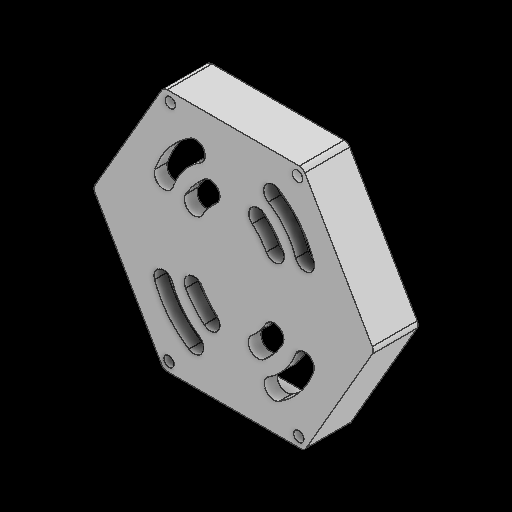
# Autodesk Inventor part: ArmPowerBoardBack
Saved by Autodesk Inventor 2025.2 (Build 292293000, 293)
## iProperties
Created: 2026-06-24
Part Number: ArmPowerBoardBack
Material: Generic
Document SubType Name: Modeling
Designer: valer
Density: 1 g/cm^3
Appearance: Default
Author: valer
Autodesk Inventor part; units mm, degrees
ref_plane "YZ Plane" through (0, 0, 0) normal (1, 0, 0) x (0, 1, 0)
ref_plane "XZ Plane" through (0, 0, 0) normal (0, 1, 0) x (-1, 0, 0)
ref_plane "XY Plane" through (0, 0, 0) normal (0, 0, 1) x (1, 0, 0)
sketch "Sketch1" plane through (0, 0, 0) normal (0, 0, 1) x (1, 0, 0)
  circle A0 centre (-20.1638, -35.1051) radius 1.25 projected
  circle A1 centre (19.9556, 35.1051) radius 1.25 projected
  circle A2 centre (20.3721, -35.1051) radius 1.25 projected
  circle A3 centre (-19.7473, 35.1051) radius 1.25 projected
  arc A4 (-17.1638, -35.1051) -> (-21.6638, -32.507) centre (-20.1638, -35.1051) ccw projected
  arc A5 (-23.0299, -32.141) -> (-21.6638, -32.507) centre (-22.1638, -31.641) ccw projected
  line L0 (-23.0299, -32.141) -> (-41.5865, 0) projected
  line L1 (-41.5865, 0) -> (-22.9176, 32.3355) projected
  arc A6 (-21.4755, 32.6529) -> (-22.9176, 32.3355) centre (-22.0516, 31.8355) ccw projected
  arc A7 (-21.4755, 32.6529) -> (-16.7473, 35.1051) centre (-19.7473, 35.1051) ccw projected
  arc A8 (-15.7473, 36.1051) -> (-16.7473, 35.1051) centre (-15.7473, 35.1051) ccw projected
  line L2 (-15.7473, 36.1051) -> (15.9556, 36.1051) projected
  arc A9 (16.9556, 35.1051) -> (15.9556, 36.1051) centre (15.9556, 35.1051) ccw projected
  arc A10 (16.9556, 35.1051) -> (21.4556, 32.507) centre (19.9556, 35.1051) ccw projected
  arc A11 (22.8216, 32.141) -> (21.4556, 32.507) centre (21.9556, 31.641) ccw projected
  line L3 (22.8216, 32.141) -> (41.5865, -0.3607) projected
  line L4 (41.5865, -0.3607) -> (23.2381, -32.141) projected
  arc A12 (21.8721, -32.507) -> (23.2381, -32.141) centre (22.3721, -31.641) ccw projected
  arc A13 (21.8721, -32.507) -> (17.3721, -35.1051) centre (20.3721, -35.1051) ccw projected
  arc A14 (16.3721, -36.1051) -> (17.3721, -35.1051) centre (16.3721, -35.1051) ccw projected
  line L5 (16.3721, -36.1051) -> (-16.1638, -36.1051) projected
  arc A15 (-17.1638, -35.1051) -> (-16.1638, -36.1051) centre (-16.1638, -35.1051) ccw projected
  line L6 (-43.3185, -1) -> (-22.4732, -37.1051) projected
  arc A16 (-22.4732, -37.1051) -> (-20.7412, -38.1051) centre (-20.7412, -36.1051) ccw projected
  line L7 (-20.7412, -38.1051) -> (20.9494, -38.1051) projected
  arc A17 (20.9494, -38.1051) -> (22.6815, -37.1051) centre (20.9494, -36.1051) ccw projected
  line L8 (22.6815, -37.1051) -> (43.3185, -1.3607) projected
  arc A18 (43.3185, -1.3607) -> (43.3185, 0.6393) centre (41.5865, -0.3607) ccw projected
  line L9 (43.3185, 0.6393) -> (22.265, 37.1051) projected
  arc A19 (22.265, 37.1051) -> (20.5329, 38.1051) centre (20.5329, 36.1051) ccw projected
  line L10 (20.5329, 38.1051) -> (-20.7412, 38.1051) projected
  arc A20 (-20.7412, 38.1051) -> (-22.4732, 37.1051) centre (-20.7412, 36.1051) ccw projected
  line L11 (-22.4732, 37.1051) -> (-43.3185, 1) projected
  arc A21 (-43.3185, 1) -> (-43.3185, -1) centre (-41.5865, 0) ccw projected
  point P0 (0, 0)
extrude "Extrusion1" add sketch "Sketch1" along normal blind 10
sketch "Sketch2" plane through (0, 0, 10) normal (0, 0, 1) x (1, 0, 0)
  arc A0 (19.392, 12.5813) -> (25.0985, 14.4351) centre (22.2452, 13.5082) ccw projected
  arc A1 (19.392, 12.5813) -> (10.8356, 23.4883) centre (0.2256, 6.3551) ccw projected
  arc A2 (13.9946, 28.5893) -> (10.8356, 23.4883) centre (12.4151, 26.0388) ccw projected
  arc A3 (25.0985, 14.4351) -> (13.9946, 28.5893) centre (0.2256, 6.3551) ccw projected
  arc A4 (-19.0054, -13.2092) -> (-24.656, -15.2268) centre (-21.8307, -14.218) ccw projected
  arc A5 (-19.0054, -13.2092) -> (-10.7215, -23.5712) centre (0.1909, -6.3551) ccw projected
  arc A6 (-13.9337, -28.639) -> (-10.7215, -23.5712) centre (-12.3276, -26.1051) ccw projected
  arc A7 (-24.656, -15.2268) -> (-13.9337, -28.639) centre (0.1909, -6.3551) ccw projected
  arc A8 (10.216, 9.6769) -> (15.4555, 12.6005) centre (12.8358, 11.1387) ccw projected
  arc A9 (10.216, 9.6769) -> (5.8047, 15.0962) centre (-7.382, -0.1428) ccw projected
  arc A10 (9.7308, 19.6334) -> (5.8047, 15.0962) centre (7.7677, 17.3648) ccw projected
  arc A11 (15.4555, 12.6005) -> (9.7308, 19.6334) centre (-7.382, -0.1428) ccw projected
  arc A12 (-5.3056, 15.1266) -> (-9.2069, 19.6851) centre (-7.2562, 17.4058) ccw projected
  arc A13 (-5.3056, 15.1266) -> (-9.7465, 9.7314) centre (7.7976, -0.1843) ccw projected
  arc A14 (-14.9699, 12.6837) -> (-9.7465, 9.7314) centre (-12.3582, 11.2076) ccw projected
  arc A15 (-9.2069, 19.6851) -> (-14.9699, 12.6837) centre (7.7976, -0.1843) ccw projected
  arc A16 (-9.7465, -9.7314) -> (-14.9699, -12.6837) centre (-12.3582, -11.2076) ccw projected
  arc A17 (-9.7465, -9.7314) -> (-5.3056, -15.1266) centre (7.7976, 0.1843) ccw projected
  arc A18 (-9.2069, -19.6851) -> (-5.3056, -15.1266) centre (-7.2562, -17.4058) ccw projected
  arc A19 (-14.9699, -12.6837) -> (-9.2069, -19.6851) centre (7.7976, 0.1843) ccw projected
  arc A20 (5.6394, -15.1565) -> (9.5156, -19.7363) centre (7.5775, -17.4464) ccw projected
  arc A21 (5.6394, -15.1565) -> (10.1097, -9.7857) centre (-7.3799, 0.2258) ccw projected
  arc A22 (15.3169, -12.7664) -> (10.1097, -9.7857) centre (12.7133, -11.2761) ccw projected
  arc A23 (9.5156, -19.7363) -> (15.3169, -12.7664) centre (-7.3799, 0.2258) ccw projected
  arc A24 (11.009, -23.6306) -> (14.1935, -28.7158) centre (12.6012, -26.1732) ccw projected
  arc A25 (11.009, -23.6306) -> (19.3494, -13.314) centre (0.1909, -6.3551) ccw projected
  arc A26 (24.9889, -15.3625) -> (19.3494, -13.314) centre (22.1691, -14.3383) ccw projected
  arc A27 (14.1935, -28.7158) -> (24.9889, -15.3625) centre (0.1909, -6.3551) ccw projected
  arc A28 (-10.2906, 23.546) -> (-13.4216, 28.6643) centre (-11.8561, 26.1051) ccw projected
  arc A29 (-10.2906, 23.546) -> (-18.9065, 12.686) centre (0.2256, 6.3551) ccw projected
  arc A30 (-24.6027, 14.5709) -> (-18.9065, 12.686) centre (-21.7546, 13.6284) ccw projected
  arc A31 (-13.4216, 28.6643) -> (-24.6027, 14.5709) centre (0.2256, 6.3551) ccw projected
  circle A32 centre (-19.7473, 35.1051) radius 1.25 construction
  circle A33 centre (20.3721, -35.1051) radius 1.25 construction
  circle A34 centre (19.9556, 35.1051) radius 1.25 construction
  circle A35 centre (-20.1638, -35.1051) radius 1.25 construction
  line L0 (-43.1103, 0.6393) -> (-22.0567, 37.1051) construction
  arc A36 (-43.1103, 0.6393) -> (-43.1103, -1.3607) centre (-41.3782, -0.3607) ccw construction
  line L1 (-22.4732, -37.1051) -> (-43.1103, -1.3607) construction
  arc A37 (-22.4732, -37.1051) -> (-20.7412, -38.1051) centre (-20.7412, -36.1051) ccw construction
  line L2 (20.9494, -38.1051) -> (-20.7412, -38.1051) construction
  arc A38 (20.9494, -38.1051) -> (22.6815, -37.1051) centre (20.9494, -36.1051) ccw construction
  line L3 (43.5268, -1) -> (22.6815, -37.1051) construction
  arc A39 (43.5268, -1) -> (43.5268, 1) centre (41.7947, 0) ccw construction
  line L4 (22.6815, 37.1051) -> (43.5268, 1) construction
  arc A40 (22.6815, 37.1051) -> (20.9494, 38.1051) centre (20.9494, 36.1051) ccw construction
  line L5 (-20.3247, 38.1051) -> (20.9494, 38.1051) construction
  arc A41 (-20.3247, 38.1051) -> (-22.0567, 37.1051) centre (-20.3247, 36.1051) ccw construction
  arc A42 (-22.4732, -37.1051) -> (-20.7412, -38.1051) centre (-20.7412, -36.1051) ccw projected
  line L6 (-20.7412, -38.1051) -> (20.9494, -38.1051) projected
  arc A43 (20.9494, -38.1051) -> (22.6815, -37.1051) centre (20.9494, -36.1051) ccw projected
  line L7 (22.6815, -37.1051) -> (43.3185, -1.3607) projected
  arc A44 (43.3185, -1.3607) -> (43.3185, 0.6393) centre (41.5865, -0.3607) ccw projected
  line L8 (43.3185, 0.6393) -> (22.265, 37.1051) projected
  arc A45 (22.265, 37.1051) -> (20.5329, 38.1051) centre (20.5329, 36.1051) ccw projected
  line L9 (20.5329, 38.1051) -> (-20.7412, 38.1051) projected
  arc A46 (-20.7412, 38.1051) -> (-22.4732, 37.1051) centre (-20.7412, 36.1051) ccw projected
  line L10 (-22.4732, 37.1051) -> (-43.3185, 1) projected
  arc A47 (-43.3185, 1) -> (-43.3185, -1) centre (-41.5865, 0) ccw projected
  line L11 (-43.3185, -1) -> (-22.4732, -37.1051) projected
  line L12 (16.3721, -36.1051) -> (-16.1638, -36.1051) projected
  arc A48 (-17.1638, -35.1051) -> (-16.1638, -36.1051) centre (-16.1638, -35.1051) ccw projected
  arc A49 (-17.1638, -35.1051) -> (-21.6638, -32.507) centre (-20.1638, -35.1051) ccw projected
  arc A50 (-23.0299, -32.141) -> (-21.6638, -32.507) centre (-22.1638, -31.641) ccw projected
  line L13 (-23.0299, -32.141) -> (-41.5865, 0) projected
  line L14 (-41.5865, 0) -> (-22.9176, 32.3355) projected
  arc A51 (-21.4755, 32.6529) -> (-22.9176, 32.3355) centre (-22.0516, 31.8355) ccw projected
  arc A52 (-21.4755, 32.6529) -> (-16.7473, 35.1051) centre (-19.7473, 35.1051) ccw projected
  arc A53 (-15.7473, 36.1051) -> (-16.7473, 35.1051) centre (-15.7473, 35.1051) ccw projected
  line L15 (-15.7473, 36.1051) -> (15.9556, 36.1051) projected
  arc A54 (16.9556, 35.1051) -> (15.9556, 36.1051) centre (15.9556, 35.1051) ccw projected
  arc A55 (16.9556, 35.1051) -> (21.4556, 32.507) centre (19.9556, 35.1051) ccw projected
  arc A56 (22.8216, 32.141) -> (21.4556, 32.507) centre (21.9556, 31.641) ccw projected
  line L16 (22.8216, 32.141) -> (41.5865, -0.3607) projected
  line L17 (41.5865, -0.3607) -> (23.2381, -32.141) projected
  arc A57 (21.8721, -32.507) -> (23.2381, -32.141) centre (22.3721, -31.641) ccw projected
  arc A58 (21.8721, -32.507) -> (17.3721, -35.1051) centre (20.3721, -35.1051) ccw projected
  arc A59 (16.3721, -36.1051) -> (17.3721, -35.1051) centre (16.3721, -35.1051) ccw projected
  circle A60 centre (-19.7473, 35.1051) radius 1.25 projected
  circle A61 centre (20.3721, -35.1051) radius 1.25 projected
  circle A62 centre (19.9556, 35.1051) radius 1.25 projected
  circle A63 centre (-20.1638, -35.1051) radius 1.25 projected
  point P0 (0, 0)
  dimension "d4" = 2.5
  measures "d4" diameter of A32
extrude "Extrusion2" add sketch "Sketch2" along normal blind 4 contours L11 A47 L10 A46 L9 A45 L8 A44 L7 A43 L6 A42 | L12 A48 A49 A50 L13 L14 A51 A52 A53 L15 A54 A55 A56 L16 L17 A57 A58 A59
sketch "Sketch3" plane through (0, 0, 14) normal (0, 0, 1) x (1, 0, 0)
  circle A0 centre (-19.7473, 35.1051) radius 1.25 construction
  circle A1 centre (19.9556, 35.1051) radius 1.25 construction
  circle A2 centre (-20.1638, -35.1051) radius 1.25 construction
  circle A3 centre (20.3721, -35.1051) radius 1.25 construction
  circle A4 centre (-19.7473, 35.1051) radius 1.6
  circle A5 centre (19.9556, 35.1051) radius 1.6
  circle A6 centre (-20.1638, -35.1051) radius 1.6
  circle A7 centre (20.3721, -35.1051) radius 1.6
  point P0 (0, 0)
  dimension "d5" = 3.2
  constraints: 4 centre point, 4 coincident, 3 equal radius
  measures "d5" diameter of A4
extrude "Extrusion3" cut sketch "Sketch3" against normal through all
body "Solid1"
